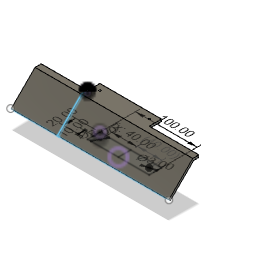
Front Shield v12 (Autodesk Fusion 360 design; units mm, degrees)
Autodesk Fusion 360 part; units mm, degrees
sketch "Attacher" plane through (0, 0, 0) normal (0, 1, 0) x (1, 0, 0)
  line L0 (0, 0) -> (100, 0)
  line L1 (100, 0) -> (100, -20)
  line L2 (100, -20) -> (0, -20)
  line L3 (0, -20) -> (0, 0)
  circle A0 centre (10, -10) radius 1.5
  line L4 (50, -20) -> (50, 0)
  circle A1 centre (90, -10) radius 1.5
  point P0 (90, -10)
  dimension "d1" = 100
  dimension "d2" = 20
  dimension "d3" = 3
  dimension "d4" = 40
  dimension "d5" = 3
  dimension "d6" = 40
  dimension "d7" = 10
  constraint horizontal L0
  constraint vertical L1
  constraint horizontal L2
  constraint vertical L3
  constraint coincident L0.start L3.end
  constraint midpoint L2 L4.start
  constraint midpoint L0 L4.end
  constraint symmetric A0.centre L4 P0
  constraint coincident P0 A1.centre
  measures "d1" distance of L1.end L2.end
  measures "d2" distance of L0.start L2.end
  measures "d3" diameter of A0
  measures "d4" distance of A0.centre L4
  measures "d5" diameter of A1
  measures "d6" distance of L4 P0
  measures "d7" distance of L2 A0.centre
extrude "Extrude1" add sketch "Attacher" along normal blind 3.5 contours L0 L2 L3 L4 makes body 1
extrude "Extrude2" add sketch "Attacher" along normal blind 3.5 contours L0 L1 L2 L4 bodies 1
move_body "Move1" bodies 1 to x (1, 0, 0) y (0, 1, 0) z (0, 0, 1) at (0, 15, 0)
move_body "Move2" bodies 1 to x (1, 0, 0) y (0, 1, 0) z (0, 0, 1) at (0, 50, 0)
sketch "FrontShield" plane through (0, 0, 0) normal (1, 0, 0) x (0, 0, -1)
  line L0 (-20, 68.5) -> (-30, 68.5)
  line L1 (-30, 68.5) -> (-68.8909, 29.6091)
  line L2 (-68.8909, 29.6091) -> (-66.416, 27.1343)
  line L3 (-66.416, 27.1343) -> (-28.5503, 65)
  line L4 (-28.5503, 65) -> (-20, 65)
  line L5 (-20, 68.5) -> (-20, 65)
  line L6 (-66.416, 27.1343, 0) -> (-66.416, 27.1343, 100)
  line L7 (-66.416, 27.1343, 0) -> (-66.416, 27.1343, -78.5)
  line L8 (-66.416, 27.1343, 100) -> (-66.416, 27.1343, 178.5)
  point P0 (-20, 68.5)
  point P1 (-20, 65)
  point P2 (-20, 0)
  dimension "d12" = 10
  dimension "d14" = 135
  dimension "d15" = 3.5
  dimension "d18" = 55
  dimension "d24" = 100
  dimension "d25" = 78.5
  dimension "d26" = 78.5
  constraint coincident P0 L0.start
  constraint perpendicular L1 L2
  constraint perpendicular L2 L3
  constraint coincident P1 L4.end
  constraint parallel L0 L4
  constraint perpendicular L4 L5
  measures "d12" distance of P0 L0.end
  measures "d14" angle of L0 L1
  measures "d15" distance of L1.end L2.end
  measures "d18" distance of L0.end L1.end
  measures "d24" distance of L2.end L3.start
  measures "d25" distance of L2.end L3.start
  measures "d26" distance of L2.end L3.start
extrude "Extrude5" add sketch "FrontShield" along normal blind 150 bodies 1
extrude "Extrude6" add sketch "FrontShield" against normal blind 50 bodies 1
copy_body "Body->Comp1" bodies 1 removing the originals makes body 2 in component "Shield"
extrude "Extrude1'" add 1 faces at (-50, 54.3697, 42.4804) along direction (-1, 0, 0) blind 25 on bodies 2 bodies 2 in component "Shield"
extrude "Extrude2'" add 1 faces at (150, 54.3697, 42.4804) along direction (1, 0, 0) blind 25 on bodies 2 bodies 2 in component "Shield"
extrude "Extrude3" add 1 faces at (-75, 54.3697, 42.4804) along direction (-1, 0, 0) blind 3.5 on bodies 2 bodies 2 in component "Shield"
extrude "Extrude4" add 1 faces at (175, 54.3697, 42.4804) along direction (1, 0, 0) blind 3.5 on bodies 2 bodies 2 in component "Shield"
extrude "Extrude5'" cut 1 faces at (178.5, 54.3697, 42.4804) along direction (-1, 0, 0) blind 2.45 on bodies 2 bodies 2 in component "Shield"
extrude "Extrude6'" cut 1 faces at (-78.5, 54.3697, 42.4804) along direction (1, 0, 0) blind 2.45 on bodies 2 bodies 2 in component "Shield"
extrude "Extrude7" add 1 faces at (176.05, 54.3697, 42.4804) along direction (1, 0, 0) blind 2.45 on bodies 2 bodies 2 in component "Shield"
extrude "Extrude8" add 1 faces at (178.5, 54.3697, 42.4804) along direction (1, 0, 0) blind 1.5 on bodies 2 bodies 2 in component "Shield"
fillet "Fillet1" radius 4 1 edges at (180, 28.3717, 67.6534) on bodies 2 in component "Shield"
fillet "Fillet2" radius 4 1 edges at (-76.05, 28.3717, 67.6534) on bodies 2 in component "Shield"
delete_face "DeleteFace1" 1 faces at (178.8949, 28.8358, 66.3644) on bodies 2 in component "Shield"
extrude "Extrude9" cut 1 faces at (180, 54.3697, 42.4804) along direction (-1, 0, 0) blind 10.67 on bodies 2 bodies 2 in component "Shield"
delete_face "DeleteFace2" 1 faces at (-76.0319, 30.5188, 64.6814) on bodies 2 in component "Shield"
extrude "Extrude10" cut 1 faces at (-76.05, 54.3697, 42.4804) along direction (1, 0, 0) blind 0.682 on bodies 2 bodies 2 in component "Shield"
extrude "Extrude11" add 1 faces at (169.33, 54.3697, 42.4804) along direction (1, 0, 0) blind 11.408 on bodies 2 bodies 2 in component "Shield"
extrude "Extrude3'" [suppressed]
extrude "Extrude4'" [suppressed]
component "Shield" placed x (1, 0, 0) y (0, 1, 0) z (0, 0, 1) at (0, 0, 0)
equation "d4 = d6"
